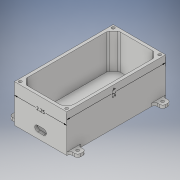
# Autodesk Inventor part: box
Saved by Autodesk Inventor 2018 (Build 220112000, 112)
## iProperties
Created: 2018-07-04
Part Number: box
Material: Generic
Document SubType Name: Modeling
Designer: Cole Tucker
Density: 1 g/cm^3
Appearance: Default
Author: Cole Tucker
Autodesk Inventor part; units mm, degrees
ref_plane "YZ Plane" through (0, 0, 0) normal (1, 0, 0) x (0, 1, 0)
ref_plane "XZ Plane" through (0, 0, 0) normal (0, 1, 0) x (-1, 0, 0)
ref_plane "XY Plane" through (0, 0, 0) normal (0, 0, 1) x (1, 0, 0)
sketch "Sketch1" plane through (0, 0, 0) normal (0, 1, 0) x (-1, 0, 0)
  line L0 (0, 0) -> (50.8, 0)
  line L1 (50.8, 0) -> (50.8, -101.6)
  line L2 (50.8, -101.6) -> (0, -101.6)
  line L3 (0, -101.6) -> (0, 0)
  dimension "d0" = 50.8
  dimension "d1" = 101.6
  constraints: 8 end point, 2 parallel, 1 horizontal, 1 perpendicular
  measures "d0" distance of L1.end L2.end
  measures "d1" distance of L0.end L1.end
extrude "Extrusion1" add sketch "Sketch1" along normal blind 3.175
sketch "Sketch2" plane through (0, 0, 0) normal (0, -1, 0) x (1, 0, 0)
  line L0 (-50.8, 0) -> (0, 0) projected
  line L1 (0, 0) -> (3.175, 0)
  line L2 (3.175, 0) -> (3.175, 3.175)
  line L3 (3.175, 3.175) -> (0, 3.175)
  line L4 (0, 3.175) -> (0, 0)
  line L5 (0, -101.6) -> (-50.8, -101.6) projected
  line L6 (-50.8, -101.6) -> (-53.975, -101.6)
  line L7 (-53.975, -101.6) -> (-53.975, -104.775)
  line L8 (-53.975, -104.775) -> (-50.8, -104.775)
  line L9 (-50.8, -104.775) -> (-50.8, -101.6)
  line L10 (3.175, 3.175) -> (-53.975, 3.175)
  line L11 (-53.975, 3.175) -> (-53.975, -104.775)
  line L12 (-53.975, -104.775) -> (3.175, -104.775)
  line L13 (3.175, -104.775) -> (3.175, 3.175)
  line L14 (-50.8, -101.6) -> (0, -101.6)
  line L15 (0, -101.6) -> (0, 0)
  line L16 (0, 0) -> (-50.8, 0)
  line L17 (-50.8, 0) -> (-50.8, -101.6)
  dimension "d4" = 3.175
  dimension "d5" = 3.175
  dimension "d6" = 3.175
  dimension "d7" = 3.175
  constraints: 32 end point, 8 parallel, 4 horizontal, 4 perpendicular
  measures "d4" distance of L3.end L2.end
  measures "d5" distance of L2.end L1.end
  measures "d6" distance of L8.end L7.end
  measures "d7" distance of L7.end L6.end
extrude "Extrusion2" add sketch "Sketch2" against normal blind 41.275 contours L17 L6 L11 L10 L4 L0 | L4 L3 L2 L1 | L1 L13 L12 L9 L5 L15 | L9 L8 L7 L6
sketch "Sketch3" plane through (0, 0, 0) normal (0, -1, 0) x (1, 0, 0)
  line L0 (0, -101.6) -> (0, 0) projected
  line L1 (3.175, 3.175) -> (3.175, -104.775) projected
  line L2 (0, 0) -> (3.175, 0)
  line L3 (3.175, 0) -> (12.065, 0)
  line L4 (12.065, 0) -> (12.065, -8.89)
  line L5 (12.065, -8.89) -> (3.175, -8.89)
  line L6 (3.175, -8.89) -> (3.175, 0)
  line L7 (-53.975, -104.775) -> (-53.975, 3.175) projected
  line L8 (-53.975, 0) -> (-62.865, 0)
  line L9 (-62.865, 0) -> (-62.865, -8.89)
  line L10 (-62.865, -8.89) -> (-53.975, -8.89)
  line L11 (-53.975, -8.89) -> (-53.975, 0)
  line L12 (-53.975, -101.6) -> (-62.865, -101.6)
  line L13 (-62.865, -101.6) -> (-62.865, -92.71)
  line L14 (-62.865, -92.71) -> (-53.975, -92.71)
  line L15 (-53.975, -92.71) -> (-53.975, -101.6)
  line L16 (3.175, -101.6) -> (12.065, -101.6)
  line L17 (12.065, -101.6) -> (12.065, -92.71)
  line L18 (12.065, -92.71) -> (3.175, -92.71)
  line L19 (3.175, -92.71) -> (3.175, -101.6)
  dimension "d11" = 8.89
  dimension "d12" = 8.89
  dimension "d13" = 8.89
  dimension "d14" = 8.89
  dimension "d15" = 8.89
  dimension "d16" = 8.89
  dimension "d17" = 8.89
  dimension "d18" = 8.89
  constraints: 34 end point, 8 parallel, 6 point on line, 5 horizontal, 4 perpendicular
  measures "d11" distance of L4.end L5.end
  measures "d12" distance of L3.end L4.end
  measures "d13" distance of L10.end L9.end
  measures "d14" distance of L9.end L8.end
  measures "d15" distance of L13.end L14.end
  measures "d16" distance of L12.end L13.end
  measures "d17" distance of L18.end L17.end
  measures "d18" distance of L17.end L16.end
extrude "Extrusion3" add sketch "Sketch3" against normal blind 3.175
fillet "Fillet1" radius 3.175 16 edges at (3.175, 1.5875, 0) (12.065, 1.5875, 0) (12.065, 1.5875, -8.89) (3.175, 1.5875, -8.89) (12.065, 1.5875, -92.71) (3.175, 1.5875, -92.71) (12.065, 1.5875, -101.6) (3.175, 1.5875, -101.6) (-53.975, 1.5875, -101.6) (-62.865, 1.5875, -101.6) (-62.865, 1.5875, -92.71) (-53.975, 1.5875, -92.71) (-53.975, 1.5875, 0) (-62.865, 1.5875, 0) (-62.865, 1.5875, -8.89) (-53.975, 1.5875, -8.89)
sketch "Sketch4" plane through (0, 3.175, 0) normal (0, 1, 0) x (1, 0, 0)
  line L0 (-59.69, 8.89) -> (-57.15, 8.89) construction
  line L1 (-58.42, 8.89) -> (-58.42, 0) construction
  line L2 (-59.69, 0) -> (-57.15, 0) construction
  line L3 (6.35, 8.89) -> (8.89, 8.89) construction
  line L4 (7.62, 8.89) -> (7.62, 0) construction
  line L5 (8.89, 0) -> (6.35, 0) construction
  line L6 (8.89, 101.6) -> (6.35, 101.6) construction
  line L7 (7.62, 101.6) -> (7.62, 92.71) construction
  line L8 (6.35, 92.71) -> (8.89, 92.71) construction
  line L9 (-57.15, 101.6) -> (-59.69, 101.6) construction
  line L10 (-58.42, 101.6) -> (-58.42, 92.71) construction
  line L11 (-59.69, 92.71) -> (-57.15, 92.71) construction
  point P0 (0, 0)
  point P1 (-58.42, 97.155)
  point P2 (7.62, 97.155)
  point P3 (7.62, 4.445)
  point P4 (-58.42, 4.445)
  constraints: 12 midpoint, 8 end point
hole "Hole1" at (-58.42, 3.175, -97.155) at (7.62, 3.175, -97.155) at (7.62, 3.175, -4.445) at (-58.42, 3.175, -4.445) direction (0, -1, 0) diameter 3.175 depth 25.4 tip angle 118
sketch "Sketch5" plane through (0, 41.275, 0) normal (0, 1, 0) x (1, 0, 0)
  line L0 (-53.975, 104.775) -> (3.175, 104.775) projected
  line L1 (3.175, 104.775) -> (-9.525, 104.775)
  arc A0 (3.175, 104.775) -> (6.35, 101.6) centre (6.35, 104.775) ccw projected
  line L2 (3.175, 104.775) -> (3.175, 92.075)
  line L3 (3.175, 92.075) -> (-9.525, 104.775)
  line L4 (3.175, -3.175) -> (-53.975, -3.175) projected
  line L5 (3.175, -3.175) -> (3.175, 9.525)
  line L6 (3.175, -3.175) -> (3.175, 12.065) projected
  line L7 (3.175, -3.175) -> (-9.525, -3.175)
  line L8 (-9.525, -3.175) -> (3.175, 9.525)
  line L9 (-25.4, 104.775) -> (-25.4, -3.175) construction
  line L10 (3.175, 104.775) -> (-53.975, 104.775)
  line L11 (-53.975, 104.775) -> (-41.275, 104.775)
  line L12 (-53.975, 104.775) -> (-53.975, 92.075)
  line L13 (-53.975, 92.075) -> (-41.275, 104.775)
  line L14 (-53.975, -3.175) -> (3.175, -3.175)
  line L15 (-53.975, -3.175) -> (-53.975, 9.525)
  line L16 (-53.975, -3.175) -> (-41.275, -3.175)
  line L17 (-41.275, -3.175) -> (-53.975, 9.525)
  point P0 (0, 0)
  dimension "d29" = 12.7
  dimension "d30" = 12.7
  dimension "d31" = 12.7
  dimension "d32" = 12.7
  constraints: 30 end point, 8 symmetric about line, 5 point on line, 2 midpoint, 1 tangent, 1 vertical
  measures "d29" distance of L0.end L1.end
  measures "d30" distance of L0.end L2.end
  measures "d31" distance of L4.start L5.end
  measures "d32" distance of L4.start L7.end
extrude "Extrusion4" add sketch "Sketch5" against normal blind 39.37
fillet "Fillet2" radius 3.175 8 edges at (-6.35, 22.225, -101.6) (0, 22.225, -95.25) (-44.45, 22.225, -101.6) (-50.8, 22.225, -95.25) (-50.8, 22.225, -6.35) (-44.45, 22.225, 0) (-6.35, 22.225, 0) (0, 22.225, -6.35)
sketch "Sketch6" plane through (0, 41.275, 0) normal (0, 1, 0) x (1, 0, 0)
  line L0 (-50.8, 93.9349) -> (-50.8, 7.6651) projected
  line L1 (0, 0) -> (0, 93.9349) projected
  point P0 (-50.8, 0)
  point P1 (-50.8, 101.6)
  point P2 (-50.8, 101.6)
  point P3 (0, 101.6)
  constraints: 2 coincident
hole "Hole2" at (0, 41.275, 0) at (-50.8, 41.275, 0) at (-50.8, 41.275, -101.6) at (0, 41.275, -101.6) direction (0, -1, 0) diameter 3.175 depth 9.525 tip angle 118
sketch "Sketch7" plane through (-53.975, 41.275, 3.175) normal (0, 0, 1) x (1, 0, 0)
  line L0 (46.3099, -38.1) -> (10.8401, -38.1) construction
  line L1 (28.575, -38.1) -> (28.575, -31.75) construction
  line L2 (28.575, -31.75) -> (25.4, -31.75) construction
  line L3 (28.575, -31.75) -> (31.75, -31.75) construction
  circle A0 centre (25.4, -31.75) radius 3.175
  circle A1 centre (31.75, -31.75) radius 3.175
  line L4 (25.4, -28.575) -> (31.75, -28.575)
  line L5 (25.4, -34.925) -> (31.75, -34.925)
  point P0 (53.975, -41.275)
  dimension "d49" = 6.35
  dimension "d50" = 3.175
  dimension "d51" = 3.175
  dimension "d52" = 6.35
  dimension "d53" = 6.35
  constraints: 10 end point, 4 point on circle, 2 centre point, 2 coincident, 2 horizontal, 2 tangent, 1 midpoint, 1 parallel, 1 perpendicular, 1 vertical
  measures "d49" distance of L1.start L1.end
  measures "d50" distance of L1.end L2.end
  measures "d51" distance of L1.end L3.end
  measures "d52" diameter of A0
  measures "d53" diameter of A1
extrude "Extrusion5" cut sketch "Sketch7" against normal blind 25.4
body "Solid1"
